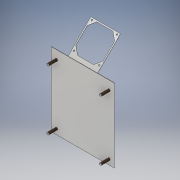
# Autodesk Inventor part: XGEN_hotbed-pcb
Saved by Autodesk Inventor 2019 (Build 230136000, 136)
## iProperties
Created: 2019-02-28
Part Number: XGEN_hotbed-pcb
Material: Generic
Document SubType Name: Sheet Metal
Designer: Rene
Density: 1 g/cm^3
Sheet Metal Rule: Default_mm
Appearance: Aluminum - Polished
Author: Rene
Autodesk Inventor part; units mm, degrees
ref_plane "YZ Plane" through (0, 0, 0) normal (1, 0, 0) x (0, 1, 0)
ref_plane "XZ Plane" through (0, 0, 0) normal (0, 1, 0) x (-1, 0, 0)
ref_plane "XY Plane" through (0, 0, 0) normal (0, 0, 1) x (1, 0, 0)
sketch "Sketch1" plane through (0, 0, 0) normal (0, 0, 1) x (1, 0, 0)
  line L0 (-90, -105) -> (90, -105)
  line L1 (90, -105) -> (90, 105)
  line L2 (-90, 105) -> (-90, -105)
  line L3 (42, 105) -> (42, 105)
  line L4 (42, 105) -> (-42, 105)
  line L5 (-42, 105) -> (-42, 105)
  line L6 (90, 105) -> (42, 105)
  line L7 (-42, 105) -> (-90, 105)
  point P0 (0, 0)
  dimension "d0" = 180
  dimension "d1" = 210
  dimension "d2" = 105
  dimension "d3" = 90
  dimension "d22" = 0
  dimension "d24" = 42
  dimension "d26" = 84
  dimension "d28" = 0
  dimension "d29" = 210
  dimension "d30" = 48
  dimension "d31" = 48
  measures "d0" distance of L0.start L0.end
  measures "d1" distance of L2.start L0.start
  measures "d2" vertical distance of point (0, 0) L0.start
  measures "d3" horizontal distance of point (0, 0) L0.start
  measures "d22" distance of L4.end L5.end
  measures "d24" horizontal distance of point (0, 0) L4.end
  measures "d26" distance of L3.end L4.end
  measures "d28" distance of L3.start L3.end
  measures "d29" distance of L0.end L1.end
  measures "d30" distance of L5.end L2.start
  measures "d31" distance of L1.end L3.start
extrude "Plate1" add sketch "Sketch1" along normal blind 0.5
sketch "Sketch6" plane through (90, 104.6464, 0.1464) normal (0, 0.7071068, 0.7071068) x (-1, 0, 0)
  line L0 (180, 0) -> (0, 0)
  line L1 (0, 0) -> (0, -92)
  line L2 (0, -92) -> (180, -92)
  line L3 (180, -92) -> (180, 0)
  constraints: 6 end point, 1 horizontal, 1 perpendicular, 1 vertical
edge flange "Flange1" height 92 angle 45 thickness 0.5 bend radius 0.5 thickness toward (0, 0.7071068, 0.7071068) relief straight relief width 0.5 relief depth 0.25 corner gap 0.5 corner form 0 edges at (-66, 105, 0) (0, 105, 0) (66, 105, 0) wall of the first edge with corners at (-90, 104.6464, 0.1464) (90, 104.6464, 0.1464) (90, 169.7003, -64.9074) (-90, 169.7003, -64.9074)
bend "Bend1"
corner "Corner1"
sketch "Sketch7" plane through (90, 169.7003, -64.9074) normal (0, -0.7071068, -0.7071068) x (-1, 0, 0)
  line L0 (180, 0) -> (0, 0) projected
  line L1 (180, -91.9393) -> (0, -91.9393) projected
  line L2 (180, -91.5858) -> (180, 0) projected
  line L3 (0, -91.5858) -> (0, 0) projected
  line L4 (0, -91.5858) -> (180, -91.5858) projected
  line L5 (0, -91.5858) -> (180, -91.5858) projected
  line L6 (180, -91.5858) -> (180, 0) projected
  line L7 (180, 0) -> (0, 0) projected
  line L8 (0, -91.5858) -> (0, 0) projected
  line L9 (0, -91.5858) -> (48, -91.5858)
  line L10 (48, -91.5858) -> (48, 0)
  line L11 (48, 0) -> (0, 0)
  line L12 (0, 0) -> (0, -91.5858)
  point P0 (90, -165.8927)
  dimension "d88" = 180
  dimension "d89" = 48
  constraints: 8 end point, 2 parallel, 1 horizontal, 1 perpendicular, 1 point on line
  measures "d88" distance of L0.start L0.end
  measures "d89" distance between parallel lines of L10 L3
extrude "Extrusion4" cut sketch "Sketch7" against normal blind 10 contours L10 L4 L3 L0
mirror "Mirror1" about plane through (0, 0, 0) normal (1, 0, 0) of "Extrusion4"
sketch "Sketch8" plane through (42, 169.7003, -64.9074) normal (0, -0.7071068, -0.7071068) x (-1, 0, 0)
  line L0 (81, -3) -> (3, -3)
  line L1 (3, -3) -> (3, -81)
  line L2 (3, -81) -> (81, -81)
  line L3 (81, -81) -> (81, -3)
  line L4 (81, -3) -> (3, -81) construction
  line L5 (3, -3) -> (81, -81) construction
  line L6 (84, 0) -> (0, 0) projected
  point P0 (42, -165.8927)
  point P1 (42, -42)
  dimension "d92" = 78
  dimension "d93" = 0
  dimension "d94" = 3
  dimension "d111" = 78
  constraints: 12 end point, 2 midpoint, 2 parallel, 1 horizontal, 1 perpendicular
  measures "d92" distance of L0.end L1.end
  measures "d93" horizontal distance of point (42, -165.893) point (42, -42)
  measures "d94" distance between parallel lines of L6 L0
  measures "d111" distance of L1.end L2.end
extrude "Extrusion5" cut sketch "Sketch8" against normal blind 10
chamfer "Chamfer2" distance 16 angle 45 4 edges at (39, 112.6014, -7.455) (39, 167.7557, -62.6093) (-39, 167.7557, -62.6093) (-39, 112.6014, -7.455)
sketch "Sketch9" plane through (42, 169.7003, -64.9074) normal (0, -0.7071068, -0.7071068) x (-1, 0, 0)
  line L0 (77.75, -5) -> (6.25, -5) construction
  line L1 (6.25, -5) -> (6.25, -76.5) construction
  line L2 (6.25, -76.5) -> (77.75, -76.5) construction
  line L3 (77.75, -76.5) -> (77.75, -5) construction
  line L4 (77.75, -5) -> (6.25, -76.5) construction
  line L5 (6.25, -5) -> (77.75, -76.5) construction
  line L6 (84, 0) -> (0, 0) construction
  point P0 (42, -165.8927)
  point P1 (42, -40.75)
  dimension "d100" = 71.5
  dimension "d101" = 71.5
  dimension "d102" = 35.75
  dimension "d103" = 5
  constraints: 12 end point, 4 coincident, 2 midpoint, 2 parallel, 1 horizontal, 1 perpendicular
  measures "d100" distance of L0.end L1.end
  measures "d101" distance of L1.end L2.end
  measures "d102" horizontal distance of point (42, -165.893) L1.end
  measures "d103" distance from line of L0.end L6
hole "Hole3" at (35.75, 166.1647, -61.3718) at (-35.75, 166.1647, -61.3718) at (-35.75, 115.6066, -10.8137) at (35.75, 115.6066, -10.8137) direction (0, 0.7071068, 0.7071068) diameter 4.2 end through all
sketch "Sketch10" plane through (0, 0, 0) normal (0, 0, -1) x (-1, 0, 0)
  line L0 (-75, -90) -> (75, -90) construction
  line L1 (75, -90) -> (75, 80) construction
  line L2 (75, 80) -> (-75, 80) construction
  line L3 (-75, 80) -> (-75, -90) construction
  line L4 (-75, -90) -> (75, 80) construction
  line L5 (75, -90) -> (-75, 80) construction
  line L6 (90, -105) -> (-90, -105) projected
  point P0 (0, -5)
  point P1 (0, 0)
  dimension "d112" = 170
  dimension "d113" = 150
  dimension "d114" = 75
  dimension "d115" = 15
  constraints: 12 end point, 4 coincident, 2 midpoint, 2 parallel, 1 horizontal, 1 perpendicular
  measures "d112" distance of L2.end L0.start
  measures "d113" distance of L0.start L0.end
  measures "d114" horizontal distance of point (0, 0) L0.start
  measures "d115" distance between parallel lines of L0 L6
hole "Hole4" at (75, 80, 0) at (75, -90, 0) at (-75, -90, 0) at (-75, 80, 0) direction (0, 0, 1) diameter 4.2 end through all
sketch "Sketch11" plane through (0, 0, 0) normal (0, 0, -1) x (-1, 0, 0)
  circle A0 centre (-75, 80) radius 2.1 projected
  circle A1 centre (-75, 80) radius 3.5
  circle A2 centre (-75, -90) radius 2.1 projected
  circle A3 centre (75, -90) radius 2.1 projected
  circle A4 centre (75, 80) radius 2.1 projected
  circle A5 centre (-75, -90) radius 3.5
  circle A6 centre (75, -90) radius 3.5
  circle A7 centre (75, 80) radius 3.5
  point P0 (0, 0)
  dimension "d123" = 7
  dimension "d124" = 7
  dimension "d125" = 7
  dimension "d126" = 7
  constraints: 4 centre point, 4 coincident
  measures "d123" diameter of A1
  measures "d124" diameter of A5
  measures "d125" diameter of A6
  measures "d126" diameter of A7
extrude "Extrusion7" add sketch "Sketch11" against normal blind 25
equation "\"d111\" = d92"
equation "\"d101\" = d100"
equation "\"d102\" = 0.5 * d101"
equation "\"d109\" = Thickness"
equation "\"d114\" = 0.5 * d113"
equation "\"d121\" = Thickness"
equation "\"d74\" = Thickness"
equation "\"d75\" = BendReliefWidth"
equation "\"d76\" = BendReliefDepth"
equation "\"d77\" = MinimumRemnant"
equation "\"d78\" = TransitionRadius"
equation "\"d81\" = BendRadius"
equation "\"d82\" = CornerReliefSize"
equation "\"d83\" = GapSize"
equation "\"d84\" = JacobiRadiusSize"
equation "\"d2\" = 0.5 * d1"
equation "\"d3\" = 0.5 * d0"
equation "\"d24\" = 0.5 * d26"
equation "\"BendRadius\" = Thickness"
equation "\"BendReliefWidth\" = Thickness"
equation "\"BendReliefDepth\" = 0.5 * Thickness"
equation "\"CornerReliefSize\" = 4 * Thickness"
equation "\"MinimumRemnant\" = 2 * Thickness"
equation "\"TransitionRadius\" = BendRadius"
equation "\"JacobiRadiusSize\" = BendRadius"
equation "\"GapSize\" = Thickness"
equation "\"Thickness\" = 0.5"
body "Solid2"
